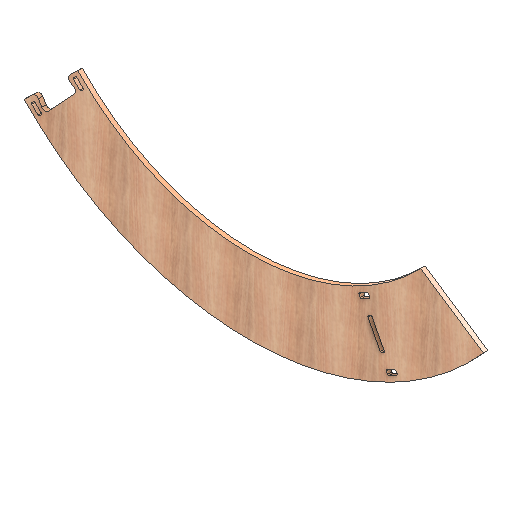
# Autodesk Inventor part: Platform D4
Saved by Autodesk Inventor 2021 (Build 250183000, 183)
## iProperties
Created: 2020-05-09
Part Number: Platform D4
Material: Wood (Birch)
Document SubType Name: Modeling
Designer: Dan Wikman
Density: 0.55 g/cm^3
Appearance: Birch - Natural Polished
Mass: 5347.46 g
Surface Area: 11725.2 cm^2
Volume: 9722.65 cm^3
Autodesk Inventor part; units mm, degrees
ref_plane "YZ Plane" through (0, 0, 0) normal (1, 0, 0) x (0, 1, 0)
ref_plane "XZ Plane" through (0, 0, 0) normal (0, 1, 0) x (-1, 0, 0)
ref_plane "XY Plane" through (0, 0, 0) normal (0, 0, 1) x (1, 0, 0)
sketch "CONTOURS" plane through (0, 0, 0) normal (0, 0, 1) x (1, 0, 0)
  arc A0 (18.8569, 427.8827) -> (1891.4893, 468.7097) centre (936.3152, 1313.2613) ccw
  line L0 (18.8569, 427.8827) -> (54.648, 462.3952)
  arc A1 (77.2131, 459.3056) -> (54.648, 462.3952) centre (64.7129, 451.9575) ccw
  line L1 (77.2131, 459.3056) -> (90.7845, 436.2188)
  arc A2 (90.7845, 436.2188) -> (115.4755, 433.495) centre (104.1468, 444.0737) ccw
  line L2 (115.4755, 433.495) -> (224.0619, 549.7797)
  arc A3 (224.0619, 549.7797) -> (220.3778, 573.8421) centre (212.7332, 560.3584) ccw
  line L3 (220.3778, 573.8421) -> (205.6826, 582.1735)
  arc A4 (202.7691, 605.2251) -> (205.6826, 582.1735) centre (212.834, 594.7873) ccw
  line L4 (202.7691, 605.2251) -> (237.5129, 638.7277)
  arc A5 (237.5129, 638.7277) -> (1635.1174, 638.7277) centre (936.3152, 1313.2613) ccw
  line L5 (1635.1174, 638.7277) -> (1891.4893, 468.7097)
  constraints: 12 end point, 12 point on circle, 6 centre point
sketch "HOLES" plane through (0, 0, 0) normal (0, 0, 1) x (1, 0, 0)
  arc A0 (75.3736, 400.9492) -> (81.0303, 400.9936) centre (78.1798, 403.7997) ccw
  line L0 (75.3736, 400.9492) -> (49.7191, 426.2049)
  arc A1 (49.6748, 431.8616) -> (49.7191, 426.2049) centre (52.5253, 429.0554) ccw
  line L1 (49.6748, 431.8616) -> (57.3918, 439.7004)
  arc A2 (63.0485, 439.7447) -> (57.3918, 439.7004) centre (60.2423, 436.8942) ccw
  line L2 (63.0485, 439.7447) -> (88.703, 414.4891)
  arc A3 (88.7473, 408.8324) -> (88.703, 414.4891) centre (85.8968, 411.6386) ccw
  line L3 (1537.9287, 212.5375) -> (1505.9814, 195.9431)
  arc A4 (1500.5879, 197.6489) -> (1505.9814, 195.9431) centre (1504.1376, 199.4928) ccw
  line L4 (1500.5879, 197.6489) -> (1495.5174, 207.4106)
  arc A5 (1497.2233, 212.8041) -> (1495.5174, 207.4106) centre (1499.0671, 209.2544) ccw
  line L5 (1497.2233, 212.8041) -> (1529.1705, 229.3985)
  arc A6 (1534.564, 227.6927) -> (1529.1705, 229.3985) centre (1531.0143, 225.8489) ccw
  line L6 (1534.564, 227.6927) -> (1539.6345, 217.931)
  arc A7 (1537.9287, 212.5375) -> (1539.6345, 217.931) centre (1536.0848, 216.0872) ccw
  line L7 (1485.873, 267.1962) -> (1476.1114, 262.1257)
  arc A8 (1470.7179, 263.8316) -> (1476.1114, 262.1257) centre (1474.2676, 265.6754) ccw
  line L8 (1470.7179, 263.8316) -> (1420.4735, 360.5606)
  arc A9 (1422.1794, 365.9541) -> (1420.4735, 360.5606) centre (1424.0232, 362.4044) ccw
  line L9 (1422.1794, 365.9541) -> (1431.9411, 371.0247)
  arc A10 (1437.3346, 369.3188) -> (1431.9411, 371.0247) centre (1433.7849, 367.475) ccw
  line L10 (1437.3346, 369.3188) -> (1487.5789, 272.5898)
  arc A11 (1485.873, 267.1962) -> (1487.5789, 272.5898) centre (1484.0292, 270.7459) ccw
  line L11 (1388.5747, 413.294) -> (1383.5041, 423.0556)
  arc A12 (1385.21, 428.4491) -> (1383.5041, 423.0556) centre (1387.0538, 424.8994) ccw
  line L12 (1385.21, 428.4491) -> (1417.1572, 445.0436)
  arc A13 (1422.5507, 443.3377) -> (1417.1572, 445.0436) centre (1419.001, 441.4939) ccw
  line L13 (1422.5507, 443.3377) -> (1427.6212, 433.5761)
  arc A14 (1425.9154, 428.1826) -> (1427.6212, 433.5761) centre (1424.0716, 431.7322) ccw
  line L14 (1425.9154, 428.1826) -> (1393.9682, 411.5881)
  arc A15 (1388.5747, 413.294) -> (1393.9682, 411.5881) centre (1392.1243, 415.1378) ccw
  line L15 (220.1514, 605.0305) -> (227.8684, 612.8694)
  arc A16 (233.5251, 612.9137) -> (227.8684, 612.8694) centre (230.7189, 610.0632) ccw
  line L16 (233.5251, 612.9137) -> (259.1796, 587.658)
  arc A17 (259.2239, 582.0014) -> (259.1796, 587.658) centre (256.3734, 584.8075) ccw
  line L17 (259.2239, 582.0014) -> (251.5069, 574.1625)
  arc A18 (245.8502, 574.1182) -> (251.5069, 574.1625) centre (248.6564, 576.9687) ccw
  line L18 (245.8502, 574.1182) -> (220.1957, 599.3738)
  arc A19 (220.1514, 605.0305) -> (220.1957, 599.3738) centre (223.0019, 602.2243) ccw
  line L19 (543.0858, 821.5545) -> (547.6833, 831.5476)
  arc A20 (547.6833, 831.5476) -> (545.7213, 836.8533) centre (544.0494, 833.2195) ccw
  line L20 (545.7213, 836.8533) -> (513.0165, 851.8999)
  arc A21 (513.0165, 851.8999) -> (507.7108, 849.9379) centre (511.3447, 848.266) ccw
  line L21 (507.7108, 849.9379) -> (503.1133, 839.9447)
  arc A22 (503.1133, 839.9447) -> (505.0753, 834.639) centre (506.7471, 838.2729) ccw
  line L22 (505.0753, 834.639) -> (537.7801, 819.5925)
  arc A23 (537.7801, 819.5925) -> (543.0858, 821.5545) centre (539.4519, 823.2264) ccw
  line L23 (481.0423, 782.4016) -> (435.4847, 683.3788)
  arc A24 (435.4847, 683.3788) -> (437.4468, 678.0731) centre (439.1186, 681.7069) ccw
  line L24 (437.4468, 678.0731) -> (447.4399, 673.4755)
  arc A25 (447.4399, 673.4755) -> (452.7456, 675.4376) centre (449.1117, 677.1094) ccw
  line L25 (452.7456, 675.4376) -> (498.3031, 774.4603)
  arc A26 (498.3031, 774.4603) -> (496.3411, 779.766) centre (494.6693, 776.1322) ccw
  line L26 (496.3411, 779.766) -> (486.348, 784.3636)
  arc A27 (486.348, 784.3636) -> (481.0423, 782.4016) centre (484.6762, 780.7297) ccw
  line L27 (446.1185, 610.7891) -> (441.521, 600.7959)
  arc A28 (436.2153, 598.8339) -> (441.521, 600.7959) centre (437.8871, 602.4678) ccw
  line L28 (436.2153, 598.8339) -> (403.5105, 613.8804)
  arc A29 (401.5485, 619.1861) -> (403.5105, 613.8804) centre (405.1824, 617.5143) ccw
  line L29 (401.5485, 619.1861) -> (406.1461, 629.1793)
  arc A30 (411.4518, 631.1413) -> (406.1461, 629.1793) centre (409.7799, 627.5074) ccw
  line L30 (411.4518, 631.1413) -> (444.1565, 616.0948)
  arc A31 (446.1185, 610.7891) -> (444.1565, 616.0948) centre (442.4847, 612.4609) ccw
  line L31 (88.7473, 408.8324) -> (81.0303, 400.9936)
  constraints: 64 end point, 64 point on circle, 32 centre point
sketch "LETTERS" plane through (0, 0, 0) normal (0, 0, 1) x (1, 0, 0)
  line L0 (228.3428, 428.6061) -> (222.1589, 433.5761)
  line L1 (222.1589, 433.5761) -> (234.7826, 448.8621)
  line L2 (234.7826, 448.8621) -> (240.0493, 444.5126)
  line L3 (240.0493, 444.5126) -> (240.1714, 444.4197)
  line L4 (240.1714, 444.4197) -> (240.2915, 444.3221)
  line L5 (240.2915, 444.3221) -> (240.4096, 444.2197)
  line L6 (240.4096, 444.2197) -> (240.5256, 444.1125)
  line L7 (240.5256, 444.1125) -> (240.6391, 444.0004)
  line L8 (240.6391, 444.0004) -> (240.7501, 443.8834)
  line L9 (240.7501, 443.8834) -> (240.8585, 443.7615)
  line L10 (240.8585, 443.7615) -> (240.9639, 443.6348)
  line L11 (240.9639, 443.6348) -> (241.0664, 443.5031)
  line L12 (241.0664, 443.5031) -> (241.1657, 443.3666)
  line L13 (228.4677, 428.5172) -> (228.3428, 428.6061)
  line L14 (228.5966, 428.4315) -> (228.4677, 428.5172)
  line L15 (228.7295, 428.3492) -> (228.5966, 428.4315)
  line L16 (228.8663, 428.2704) -> (228.7295, 428.3492)
  line L17 (229.0071, 428.1953) -> (228.8663, 428.2704)
  line L18 (229.1518, 428.1241) -> (229.0071, 428.1953)
  line L19 (229.3004, 428.0569) -> (229.1518, 428.1241)
  line L20 (229.4528, 427.9939) -> (229.3004, 428.0569)
  line L21 (229.609, 427.9352) -> (229.4528, 427.9939)
  line L22 (229.7689, 427.8809) -> (229.609, 427.9352)
  line L23 (229.9324, 427.8313) -> (229.7689, 427.8809)
  line L24 (230.0995, 427.7865) -> (229.9324, 427.8313)
  line L25 (230.2701, 427.7466) -> (230.0995, 427.7865)
  line L26 (230.444, 427.7117) -> (230.2701, 427.7466)
  line L27 (230.6212, 427.6819) -> (230.444, 427.7117)
  line L28 (230.8016, 427.6574) -> (230.6212, 427.6819)
  line L29 (230.9849, 427.6383) -> (230.8016, 427.6574)
  line L30 (231.1712, 427.6246) -> (230.9849, 427.6383)
  line L31 (231.3602, 427.6165) -> (231.1712, 427.6246)
  line L32 (231.5519, 427.6141) -> (231.3602, 427.6165)
  line L33 (231.7459, 427.6174) -> (231.5519, 427.6141)
  line L34 (231.9423, 427.6264) -> (231.7459, 427.6174)
  line L35 (232.1408, 427.6413) -> (231.9423, 427.6264)
  line L36 (232.3412, 427.662) -> (232.1408, 427.6413)
  line L37 (232.5433, 427.6887) -> (232.3412, 427.662)
  line L38 (232.747, 427.7212) -> (232.5433, 427.6887)
  line L39 (232.9521, 427.7597) -> (232.747, 427.7212)
  line L40 (233.1584, 427.8041) -> (232.9521, 427.7597)
  line L41 (233.3656, 427.8544) -> (233.1584, 427.8041)
  line L42 (233.5736, 427.9106) -> (233.3656, 427.8544)
  line L43 (233.7821, 427.9726) -> (233.5736, 427.9106)
  line L44 (233.991, 428.0404) -> (233.7821, 427.9726)
  line L45 (234.2, 428.1139) -> (233.991, 428.0404)
  line L46 (234.409, 428.193) -> (234.2, 428.1139)
  line L47 (234.6177, 428.2776) -> (234.409, 428.193)
  line L48 (234.8258, 428.3677) -> (234.6177, 428.2776)
  line L49 (235.0333, 428.4632) -> (234.8258, 428.3677)
  line L50 (235.2399, 428.5638) -> (235.0333, 428.4632)
  line L51 (235.4454, 428.6696) -> (235.2399, 428.5638)
  line L52 (235.6496, 428.7803) -> (235.4454, 428.6696)
  line L53 (235.8522, 428.8958) -> (235.6496, 428.7803)
  line L54 (236.0532, 429.0159) -> (235.8522, 428.8958)
  line L55 (236.2524, 429.1405) -> (236.0532, 429.0159)
  line L56 (236.4495, 429.2695) -> (236.2524, 429.1405)
  line L57 (236.6444, 429.4026) -> (236.4495, 429.2695)
  line L58 (236.8369, 429.5396) -> (236.6444, 429.4026)
  line L59 (237.0269, 429.6804) -> (236.8369, 429.5396)
  line L60 (237.2142, 429.8249) -> (237.0269, 429.6804)
  line L61 (237.3987, 429.9727) -> (237.2142, 429.8249)
  line L62 (237.5803, 430.1237) -> (237.3987, 429.9727)
  line L63 (237.7587, 430.2777) -> (237.5803, 430.1237)
  line L64 (237.934, 430.4346) -> (237.7587, 430.2777)
  line L65 (238.2747, 430.7559) -> (237.934, 430.4346)
  line L66 (238.6014, 431.0861) -> (238.2747, 430.7559)
  line L67 (238.9137, 431.4236) -> (238.6014, 431.0861)
  line L68 (239.2109, 431.7669) -> (238.9137, 431.4236)
  line L69 (239.4929, 432.1144) -> (239.2109, 431.7669)
  line L70 (239.7594, 432.4649) -> (239.4929, 432.1144)
  line L71 (240.0148, 432.8236) -> (239.7594, 432.4649)
  line L72 (240.2628, 433.1961) -> (240.0148, 432.8236)
  line L73 (240.5022, 433.582) -> (240.2628, 433.1961)
  line L74 (240.7316, 433.9805) -> (240.5022, 433.582)
  line L75 (240.9497, 434.3906) -> (240.7316, 433.9805)
  line L76 (241.1552, 434.8114) -> (240.9497, 434.3906)
  line L77 (241.2528, 435.0254) -> (241.1552, 434.8114)
  line L78 (241.3468, 435.2416) -> (241.2528, 435.0254)
  line L79 (241.4371, 435.4598) -> (241.3468, 435.2416)
  line L80 (241.5233, 435.68) -> (241.4371, 435.4598)
  line L81 (241.6055, 435.9017) -> (241.5233, 435.68)
  line L82 (241.6835, 436.125) -> (241.6055, 435.9017)
  line L83 (241.7571, 436.3496) -> (241.6835, 436.125)
  line L84 (241.8262, 436.5752) -> (241.7571, 436.3496)
  line L85 (241.8908, 436.8018) -> (241.8262, 436.5752)
  line L86 (241.9505, 437.0289) -> (241.8908, 436.8018)
  line L87 (242.0055, 437.2566) -> (241.9505, 437.0289)
  line L88 (242.0555, 437.4844) -> (242.0055, 437.2566)
  line L89 (242.1005, 437.7123) -> (242.0555, 437.4844)
  line L90 (242.1404, 437.9399) -> (242.1005, 437.7123)
  line L91 (242.175, 438.1671) -> (242.1404, 437.9399)
  line L92 (242.2045, 438.3936) -> (242.175, 438.1671)
  line L93 (242.2286, 438.6191) -> (242.2045, 438.3936)
  line L94 (242.2474, 438.8435) -> (242.2286, 438.6191)
  line L95 (242.2608, 439.0665) -> (242.2474, 438.8435)
  line L96 (242.2688, 439.288) -> (242.2608, 439.0665)
  line L97 (242.2714, 439.5075) -> (242.2688, 439.288)
  line L98 (242.2686, 439.7251) -> (242.2714, 439.5075)
  line L99 (242.2604, 439.9404) -> (242.2686, 439.7251)
  line L100 (242.2468, 440.1532) -> (242.2604, 439.9404)
  line L101 (242.2279, 440.3633) -> (242.2468, 440.1532)
  line L102 (242.2037, 440.5706) -> (242.2279, 440.3633)
  line L103 (242.1742, 440.7747) -> (242.2037, 440.5706)
  line L104 (242.1395, 440.9757) -> (242.1742, 440.7747)
  line L105 (242.0998, 441.1732) -> (242.1395, 440.9757)
  line L106 (242.055, 441.3671) -> (242.0998, 441.1732)
  line L107 (242.0052, 441.5573) -> (242.055, 441.3671)
  line L108 (241.9506, 441.7435) -> (242.0052, 441.5573)
  line L109 (241.8913, 441.9258) -> (241.9506, 441.7435)
  line L110 (241.8274, 442.1039) -> (241.8913, 441.9258)
  line L111 (241.759, 442.2776) -> (241.8274, 442.1039)
  line L112 (241.6862, 442.447) -> (241.759, 442.2776)
  line L113 (241.6092, 442.612) -> (241.6862, 442.447)
  line L114 (241.5281, 442.7723) -> (241.6092, 442.612)
  line L115 (241.443, 442.928) -> (241.5281, 442.7723)
  line L116 (241.3542, 443.079) -> (241.443, 442.928)
  line L117 (241.2617, 443.2252) -> (241.3542, 443.079)
  line L118 (241.1657, 443.3666) -> (241.2617, 443.2252)
  constraints: 238 end point, 3 perpendicular
extrude "Extrusion4" add sketch "CONTOURS" along normal blind 18
extrude "Extrusion5" cut sketch "HOLES" along normal blind 18 contours L0 A1 L1 A2 L2 A3 L31 A0 | L3 A4 L4 A5 L5 A6 L6 A7 | L7 A8 L8 A9 L9 A10 L10 A11 | L11 A12 L12 A13 L13 A14 L14 A15 | L15 A16 L16 A17 L17 A18 L18 A19
body "Solid3"
